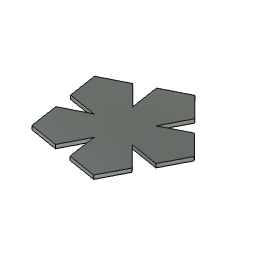
dodecahedron (Autodesk Fusion 360 design; units mm, degrees)
Autodesk Fusion 360 part; units mm, degrees
sketch "Sketch1" plane through (0, 0, 0) normal (0, 0, 1) x (1, 0, 0)
  line L0 (17.5654, 17.3955) -> (-11.1161, 22.0812)
  line L1 (-11.1161, 22.0812) -> (-24.4355, -3.7486)
  line L2 (-24.4355, -3.7486) -> (-3.9858, -24.3979)
  line L3 (-3.9858, -24.3979) -> (21.9721, -11.3301)
  line L4 (21.9721, -11.3301) -> (17.5654, 17.3955)
  line L5 (17.5654, 17.3955) -> (21.9721, -11.3301)
  line L6 (21.9721, -11.3301) -> (50.6536, -16.0158)
  line L7 (50.6536, -16.0158) -> (63.973, 9.814)
  line L8 (63.973, 9.814) -> (43.5233, 30.4633)
  line L9 (43.5233, 30.4633) -> (17.5654, 17.3955)
  line L10 (17.5654, 17.3955) -> (30.8847, 43.2253)
  line L11 (30.8847, 43.2253) -> (10.4351, 63.8746)
  line L12 (10.4351, 63.8746) -> (-15.5229, 50.8068)
  line L13 (-15.5229, 50.8068) -> (-11.1161, 22.0812)
  line L14 (-11.1161, 22.0812) -> (17.5654, 17.3955)
  line L15 (-11.1161, 22.0812) -> (-31.5658, 42.7305)
  line L16 (-31.5658, 42.7305) -> (-57.5237, 29.6627)
  line L17 (-57.5237, 29.6627) -> (-53.117, 0.937)
  line L18 (-53.117, 0.937) -> (-24.4355, -3.7486)
  line L19 (-24.4355, -3.7486) -> (-11.1161, 22.0812)
  line L20 (-24.4355, -3.7486) -> (-50.3935, -16.8164)
  line L21 (-50.3935, -16.8164) -> (-45.9867, -45.542)
  line L22 (-45.9867, -45.542) -> (-17.3052, -50.2277)
  line L23 (-17.3052, -50.2277) -> (-3.9858, -24.3979)
  line L24 (-3.9858, -24.3979) -> (-24.4355, -3.7486)
  line L25 (-3.9858, -24.3979) -> (0.4209, -53.1236)
  line L26 (0.4209, -53.1236) -> (29.1024, -57.8092)
  line L27 (29.1024, -57.8092) -> (42.4218, -31.9795)
  line L28 (42.4218, -31.9795) -> (21.9721, -11.3301)
  line L29 (21.9721, -11.3301) -> (-3.9858, -24.3979)
  point P0 (39.5375, 6.0654)
  point P1 (6.4492, 39.4767)
  point P2 (-35.5516, 18.3326)
  point P3 (-28.4213, -28.1465)
  point P4 (17.9863, -35.7281)
  dimension "d1" = 20
  measures "d1" distance of origin L4
extrude "Extrude1" add sketch "Sketch1" along normal blind 3.8
sketch "Sketch2" plane through (0, 0, 3.8) normal (0, 0, 1) x (-1, 0, 0)
  line L0 (-42.4218, 31.9795) -> (-21.9721, 11.3301)
  line L1 (-21.9721, 11.3301) -> (-50.6536, 16.0158)
  line L2 (-50.6536, 16.0158) -> (-63.973, -9.814)
  line L3 (-63.973, -9.814) -> (-43.5233, -30.4633)
  line L4 (-43.5233, -30.4633) -> (-17.5654, -17.3955)
  line L5 (-17.5654, -17.3955) -> (-30.8847, -43.2253)
  line L6 (-30.8847, -43.2253) -> (-10.4351, -63.8746)
  line L7 (-10.4351, -63.8746) -> (15.5229, -50.8068)
  line L8 (15.5229, -50.8068) -> (11.1161, -22.0812)
  line L9 (11.1161, -22.0812) -> (31.5658, -42.7305)
  line L10 (31.5658, -42.7305) -> (57.5237, -29.6627)
  line L11 (57.5237, -29.6627) -> (53.117, -0.937)
  line L12 (53.117, -0.937) -> (24.4355, 3.7486)
  line L13 (24.4355, 3.7486) -> (50.3935, 16.8164)
  line L14 (50.3935, 16.8164) -> (45.9867, 45.542)
  line L15 (45.9867, 45.542) -> (17.3052, 50.2277)
  line L16 (17.3052, 50.2277) -> (3.9858, 24.3979)
  line L17 (3.9858, 24.3979) -> (-0.4209, 53.1236)
  line L18 (-0.4209, 53.1236) -> (-29.1024, 57.8092)
  line L19 (-29.1024, 57.8092) -> (-42.4218, 31.9795)
